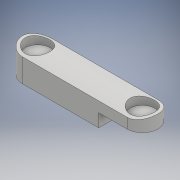
# Autodesk Inventor part: 第一臂
Saved by Autodesk Inventor 2017 (Build 210142000, 142)
## iProperties
Part Number: 第一臂
Material: 一般
Document SubType Name: Modeling
Designer: Brian
Density: 1 g/cm^3
Appearance: 預設
Author: Brian
Autodesk Inventor part; units mm, degrees
ref_plane "YZ Plane" through (0, 0, 0) normal (1, 0, 0) x (0, 1, 0)
ref_plane "XZ Plane" through (0, 0, 0) normal (0, 1, 0) x (-1, 0, 0)
ref_plane "XY Plane" through (0, 0, 0) normal (0, 0, 1) x (1, 0, 0)
sketch "草圖1" plane through (0, 0, 0) normal (0, 0, 1) x (1, 0, 0)
  circle A0 centre (0, 0) radius 17.5
  circle A1 centre (120, 0) radius 17.5
  line L0 (0, 17.5) -> (120, 17.5)
  line L1 (120, 17.5) -> (120, -17.5)
  line L2 (120, -17.5) -> (0, -17.5)
  line L3 (0, -17.5) -> (0, 17.5)
  dimension "d0" = 35
  dimension "d1" = 35
  dimension "d4" = 120
  dimension "d5" = 35
  constraints: 8 end point, 3 coincident, 2 centre point, 2 midpoint, 2 parallel, 1 horizontal, 1 perpendicular
  measures "d0" diameter of A0
  measures "d1" diameter of A1
  measures "d4" distance of L0.start L0.end
  measures "d5" distance between parallel lines of L2 L0
extrude "擠出1" add sketch "草圖1" along normal blind 15
sketch "草圖2" plane through (0, 0, 15) normal (0, 0, 1) x (1, 0, 0)
  circle A0 centre (0, 0) radius 14
  arc A1 (120, -17.5) -> (120, 17.5) centre (120, 0) ccw projected
  circle A2 centre (120, 0) radius 14
  dimension "d6" = 28
  dimension "d7" = 28
  constraints: 2 centre point, 2 coincident
  measures "d6" diameter of A2
  measures "d7" diameter of A0
extrude "擠出2" cut sketch "草圖2" against normal blind 10
sketch "草圖3" plane through (0, 0, 0) normal (1, 0, 0) x (0, 1, 0)
  circle A0 centre (0, -33.7441) radius 48.7441
  point P0 (0, 0)
  constraints: 1 centre point
extrude "擠出3" cut sketch "草圖3" along normal through all both and the other way through all keep common part
sketch "草圖5" plane through (0, 0, 0) normal (0, 0, -1) x (-1, 0, 0)
  circle A0 centre (0, 0) radius 14 projected
  line L0 (0, 17.5) -> (-120, 17.5) projected
  arc A1 (-120, 17.5) -> (-120, -17.5) centre (-120, 0) ccw projected
  line L1 (-120, -17.5) -> (0, -17.5) projected
  arc A2 (0, -17.5) -> (0, 17.5) centre (0, 0) ccw projected
  line L2 (0, 17.5) -> (-120, 17.5) projected
  line L3 (-87.5, 17.5) -> (-87.5, -17.5)
  line L4 (-120, -17.5) -> (0, -17.5) projected
  dimension "d13" = 50
  constraints: 2 end point, 2 point on line, 1 perpendicular
extrude "擠出4" add sketch "草圖5" along normal blind 15 contours A0 | A2 L1 L3 L0
